Autodesk Fusion 360 part; units mm, degrees
(part 2 of 4)
  line L504 (36.7119, 7.7268) -> (35.9792, 7.7268)
  line L505 (35.9792, 7.7268) -> (35.9792, 6.8541)
  line L506 (35.9792, 6.8541) -> (37.0036, 6.8223)
  line L507 (37.0036, 6.8223) -> (37.0474, 6.7171)
  line L508 (37.0474, 6.7171) -> (36.8838, 6.6359)
  line L509 (36.8838, 6.6359) -> (35.6903, 6.6677)
  line L510 (35.6903, 6.6677) -> (35.641, 6.745)
  line L511 (7.544, 26.4091) -> (7.544, 26.4091)
  line L512 (38.6779, 6.745) -> (38.6998, 8.9814)
  line L513 (38.6998, 8.9814) -> (38.9315, 9.0218)
  line L514 (38.9315, 9.0218) -> (39.0161, 8.9268)
  line L515 (39.0161, 8.9268) -> (38.9941, 6.6904)
  line L516 (38.9941, 6.6904) -> (38.7624, 6.65)
  line L517 (38.7624, 6.65) -> (38.6779, 6.745)
  line L518 (10.5809, 26.4091) -> (10.5809, 26.4091)
  line L519 (41.4963, 7.625) -> (41.6977, 7.7268)
  line L520 (41.6977, 7.7268) -> (41.7415, 7.8359)
  line L521 (41.7415, 7.8359) -> (41.7304, 8.6571)
  line L522 (41.7304, 8.6571) -> (41.6071, 8.7735)
  line L523 (41.6071, 8.7735) -> (41.4033, 8.8177)
  line L524 (41.4033, 8.8177) -> (40.8397, 8.8177)
  line L525 (40.8397, 8.8177) -> (40.8178, 6.6904)
  line L526 (40.8178, 6.6904) -> (40.5861, 6.65)
  line L527 (40.5861, 6.65) -> (40.5015, 6.745)
  line L528 (40.5015, 6.745) -> (40.5234, 8.9814)
  line L529 (40.5234, 8.9814) -> (40.6706, 9.0359)
  line L530 (40.6706, 9.0359) -> (41.5804, 9.0217)
  line L531 (41.5804, 9.0217) -> (41.8126, 8.9469)
  line L532 (41.8126, 8.9469) -> (41.9914, 8.8165)
  line L533 (41.9914, 8.8165) -> (42.0576, 8.7138)
  line L534 (42.0576, 8.7138) -> (42.0797, 8.5995)
  line L535 (42.0797, 8.5995) -> (42.0742, 7.7774)
  line L536 (42.0742, 7.7774) -> (42.0304, 7.6691)
  line L537 (42.0304, 7.6691) -> (41.7528, 7.4614)
  line L538 (41.7528, 7.4614) -> (42.184, 6.7123)
  line L539 (42.184, 6.7123) -> (41.9726, 6.6395)
  line L540 (41.9726, 6.6395) -> (41.8711, 6.6959)
  line L541 (41.8711, 6.6959) -> (41.3709, 7.5343)
  line L542 (41.3709, 7.5343) -> (41.4963, 7.625)
  line L543 (13.3994, 27.2891) -> (13.3994, 27.2891)
  line L544 (43.4792, 7.945) -> (44.3317, 7.9132)
  line L545 (44.3317, 7.9132) -> (44.3755, 7.8071)
  line L546 (44.3755, 7.8071) -> (44.2119, 7.7268)
  line L547 (44.2119, 7.7268) -> (43.4792, 7.7268)
  line L548 (43.4792, 7.7268) -> (43.4573, 6.6904)
  line L549 (43.4573, 6.6904) -> (43.2256, 6.65)
  line L550 (43.2256, 6.65) -> (43.141, 6.745)
  line L551 (43.141, 6.745) -> (43.1629, 8.9814)
  line L552 (43.1629, 8.9814) -> (43.3101, 9.0359)
  line L553 (43.3101, 9.0359) -> (44.5036, 9.0041)
  line L554 (44.5036, 9.0041) -> (44.5474, 8.8989)
  line L555 (44.5474, 8.8989) -> (44.3838, 8.8177)
  line L556 (44.3838, 8.8177) -> (43.4792, 8.8177)
  line L557 (43.4792, 8.8177) -> (43.4792, 7.945)
  line L558 (15.3822, 27.6091) -> (15.3822, 27.6091)
  line L559 (46.1779, 8.8177) -> (45.5921, 8.8605)
  line L560 (45.5921, 8.8605) -> (45.5702, 8.9689)
  line L561 (45.5702, 8.9689) -> (45.727, 9.0359)
  line L562 (45.727, 9.0359) -> (47.0867, 9.0041)
  line L563 (47.0867, 9.0041) -> (47.1306, 8.898)
  line L564 (47.1306, 8.898) -> (46.967, 8.8177)
  line L565 (46.967, 8.8177) -> (46.5161, 8.8177)
  line L566 (46.5161, 8.8177) -> (46.4941, 6.6904)
  line L567 (46.4941, 6.6904) -> (46.2624, 6.65)
  line L568 (46.2624, 6.65) -> (46.1779, 6.745)
  line L569 (46.1779, 6.745) -> (46.1779, 8.8177)
  line L570 (18.0809, 28.4818) -> (18.0809, 28.4818)
  line L571 (48.0029, 6.745) -> (48.0248, 8.9814)
  line L572 (48.0248, 8.9814) -> (48.2566, 9.0218)
  line L573 (48.2566, 9.0218) -> (48.3411, 8.9268)
  line L574 (48.3411, 8.9268) -> (48.3411, 7.945)
  line L575 (48.3411, 7.945) -> (49.3528, 7.945)
  line L576 (49.3528, 7.945) -> (49.3747, 8.9814)
  line L577 (49.3747, 8.9814) -> (49.6065, 9.0218)
  line L578 (49.6065, 9.0218) -> (49.691, 8.9268)
  line L579 (49.691, 8.9268) -> (49.6691, 6.6904)
  line L580 (49.6691, 6.6904) -> (49.4374, 6.65)
  line L581 (49.4374, 6.65) -> (49.3528, 6.745)
  line L582 (49.3528, 6.745) -> (49.3528, 7.7268)
  line L583 (49.3528, 7.7268) -> (48.3411, 7.7268)
  line L584 (48.3411, 7.7268) -> (48.3192, 6.6904)
  line L585 (48.3192, 6.6904) -> (48.0875, 6.65)
  line L586 (48.0875, 6.65) -> (48.0029, 6.745)
  line L587 (19.906, 26.4091) -> (19.906, 26.4091)
  line L588 (51.1779, 6.745) -> (51.1998, 8.9814)
  line L589 (51.1998, 8.9814) -> (51.4315, 9.0218)
  line L590 (51.4315, 9.0218) -> (51.5161, 8.9268)
  line L591 (51.5161, 8.9268) -> (51.4941, 6.6904)
  line L592 (51.4941, 6.6904) -> (51.2624, 6.65)
  line L593 (51.2624, 6.65) -> (51.1779, 6.745)
  line L594 (23.0809, 26.4091) -> (23.0809, 26.4091)
  line L595 (53.9963, 7.625) -> (54.1977, 7.7268)
  line L596 (54.1977, 7.7268) -> (54.2415, 7.8359)
  line L597 (54.2415, 7.8359) -> (54.2304, 8.6571)
  line L598 (54.2304, 8.6571) -> (54.1071, 8.7735)
  line L599 (54.1071, 8.7735) -> (53.9033, 8.8177)
  line L600 (53.9033, 8.8177) -> (53.3397, 8.8177)
  line L601 (53.3397, 8.8177) -> (53.3178, 6.6904)
  line L602 (53.3178, 6.6904) -> (53.0861, 6.65)
  line L603 (53.0861, 6.65) -> (53.0015, 6.745)
  line L604 (53.0015, 6.745) -> (53.0234, 8.9814)
  line L605 (53.0234, 8.9814) -> (53.1706, 9.0359)
  line L606 (53.1706, 9.0359) -> (54.0804, 9.0217)
  line L607 (54.0804, 9.0217) -> (54.3126, 8.9469)
  line L608 (54.3126, 8.9469) -> (54.4914, 8.8165)
  line L609 (54.4914, 8.8165) -> (54.5576, 8.7138)
  line L610 (54.5576, 8.7138) -> (54.5797, 8.5995)
  line L611 (54.5797, 8.5995) -> (54.5742, 7.7774)
  line L612 (54.5742, 7.7774) -> (54.5304, 7.6691)
  line L613 (54.5304, 7.6691) -> (54.2528, 7.4614)
  line L614 (54.2528, 7.4614) -> (54.684, 6.7123)
  line L615 (54.684, 6.7123) -> (54.4726, 6.6395)
  line L616 (54.4726, 6.6395) -> (54.3711, 6.6959)
  line L617 (54.3711, 6.6959) -> (53.8709, 7.5343)
  line L618 (53.8709, 7.5343) -> (53.9963, 7.625)
  line L619 (25.8994, 27.2891) -> (25.8994, 27.2891)
  line L620 (56.7485, 6.9372) -> (56.9939, 6.9257)
  line L621 (56.9939, 6.9257) -> (57.0154, 6.8218)
  line L622 (57.0154, 6.8218) -> (56.9009, 6.7411)
  line L623 (56.9009, 6.7411) -> (56.6334, 6.6527)
  line L624 (56.6334, 6.6527) -> (56.3286, 6.6399)
  line L625 (56.3286, 6.6399) -> (56.0505, 6.7001)
  line L626 (56.0505, 6.7001) -> (55.8224, 6.8302)
  line L627 (55.8224, 6.8302) -> (55.7229, 6.9399)
  line L628 (55.7229, 6.9399) -> (55.6731, 7.0628)
  line L629 (55.6731, 7.0628) -> (55.6731, 8.609)
  line L630 (55.6731, 8.609) -> (55.7229, 8.7319)
  line L631 (55.7229, 8.7319) -> (55.8224, 8.8416)
  line L632 (55.8224, 8.8416) -> (56.0505, 8.9717)
  line L633 (56.0505, 8.9717) -> (56.3286, 9.0319)
  line L634 (56.3286, 9.0319) -> (56.6334, 9.0191)
  line L635 (56.6334, 9.0191) -> (56.9009, 8.9307)
  line L636 (56.9009, 8.9307) -> (57.0271, 8.8104)
  line L637 (57.0271, 8.8104) -> (56.9064, 8.7081)
  line L638 (56.9064, 8.7081) -> (56.547, 8.8131)
  line L639 (56.547, 8.8131) -> (56.2626, 8.802)
  line L640 (56.2626, 8.802) -> (56.0828, 8.7113)
  line L641 (56.0828, 8.7113) -> (56.0087, 8.6146)
  line L642 (56.0087, 8.6146) -> (55.9946, 8.5407)
  line L643 (55.9946, 8.5407) -> (55.9982, 7.0932)
  line L644 (55.9982, 7.0932) -> (56.0511, 6.9909)
  line L645 (56.0511, 6.9909) -> (56.2125, 6.8859)
  line L646 (56.2125, 6.8859) -> (56.4905, 6.8516)
  line L647 (56.4905, 6.8516) -> (56.7485, 6.9372)
  line L648 (28.6515, 26.6013) -> (28.6515, 26.6013)
  line L649 (58.141, 6.745) -> (58.1629, 8.9814)
  line L650 (58.1629, 8.9814) -> (58.3101, 9.0359)
  line L651 (58.3101, 9.0359) -> (59.5036, 9.0041)
  line L652 (59.5036, 9.0041) -> (59.5474, 8.8989)
  line L653 (59.5474, 8.8989) -> (59.3838, 8.8177)
  line L654 (59.3838, 8.8177) -> (58.4792, 8.8177)
  line L655 (58.4792, 8.8177) -> (58.4792, 7.945)
  line L656 (58.4792, 7.945) -> (59.3317, 7.9132)
  line L657 (59.3317, 7.9132) -> (59.3755, 7.8071)
  line L658 (59.3755, 7.8071) -> (59.2119, 7.7268)
  line L659 (59.2119, 7.7268) -> (58.4792, 7.7268)
  line L660 (58.4792, 7.7268) -> (58.4792, 6.8541)
  line L661 (58.4792, 6.8541) -> (59.5036, 6.8223)
  line L662 (59.5036, 6.8223) -> (59.5474, 6.7171)
  line L663 (59.5474, 6.7171) -> (59.3838, 6.6359)
  line L664 (59.3838, 6.6359) -> (58.1903, 6.6677)
  line L665 (58.1903, 6.6677) -> (58.141, 6.745)
  line L666 (30.044, 26.4091) -> (30.044, 26.4091)
  line L667 (31.9045, 5.882) -> (31.9463, 5.7785)
  line L668 (31.9463, 5.7785) -> (31.7415, 5.703)
  line L669 (31.7415, 5.703) -> (31.4641, 5.8096)
  line L670 (31.4641, 5.8096) -> (31.1753, 5.7983)
  line L671 (31.1753, 5.7983) -> (30.9927, 5.7062)
  line L672 (30.9927, 5.7062) -> (30.9175, 5.608)
  line L673 (30.9175, 5.608) -> (30.9067, 4.0986)
  line L674 (30.9067, 4.0986) -> (30.9604, 3.9946)
  line L675 (30.9604, 3.9946) -> (31.1244, 3.8881)
  line L676 (31.1244, 3.8881) -> (31.347, 3.8507)
  line L677 (31.347, 3.8507) -> (31.7908, 3.8507)
  line L678 (31.7908, 3.8507) -> (31.7908, 4.6739)
  line L679 (31.7908, 4.6739) -> (31.4795, 4.7288)
  line L680 (31.4795, 4.7288) -> (31.4795, 4.835)
  line L681 (31.4795, 4.835) -> (31.6244, 4.8887)
  line L682 (31.6244, 4.8887) -> (32.091, 4.8466)
  line L683 (32.091, 4.8466) -> (32.1237, 4.7813)
  line L684 (32.1237, 4.7813) -> (32.1021, 3.6908)
  line L685 (32.1021, 3.6908) -> (31.9573, 3.6359)
  line L686 (31.9573, 3.6359) -> (31.2423, 3.64)
  line L687 (31.2423, 3.64) -> (30.9598, 3.7007)
  line L688 (30.9598, 3.7007) -> (30.7282, 3.8321)
  line L689 (30.7282, 3.8321) -> (30.6271, 3.9431)
  line L690 (30.6271, 3.9431) -> (30.5766, 4.0677)
  line L691 (30.5766, 4.0677) -> (30.5766, 5.6023)
  line L692 (30.5766, 5.6023) -> (30.6271, 5.7272)
  line L693 (30.6271, 5.7272) -> (30.7282, 5.8385)
  line L694 (30.7282, 5.8385) -> (30.9598, 5.9707)
  line L695 (30.9598, 5.9707) -> (31.2423, 6.0318)
  line L696 (31.2423, 6.0318) -> (31.5519, 6.0188)
  line L697 (31.5519, 6.0188) -> (31.9045, 5.882)
  line L698 (3.8076, 25.5461) -> (3.8076, 25.5461)
  line L699 (33.6779, 5.8177) -> (33.0921, 5.8605)
  line L700 (33.0921, 5.8605) -> (33.0702, 5.9689)
  line L701 (33.0702, 5.9689) -> (33.227, 6.0359)
  line L702 (33.227, 6.0359) -> (34.5867, 6.0041)
  line L703 (34.5867, 6.0041) -> (34.6306, 5.898)
  line L704 (34.6306, 5.898) -> (34.467, 5.8177)
  line L705 (34.467, 5.8177) -> (34.0161, 5.8177)
  line L706 (34.0161, 5.8177) -> (33.9941, 3.6904)
  line L707 (33.9941, 3.6904) -> (33.7624, 3.65)
  line L708 (33.7624, 3.65) -> (33.6779, 3.745)
  line L709 (33.6779, 3.745) -> (33.6779, 5.8177)
  line L710 (5.5809, 25.4818) -> (5.5809, 25.4818)
  line L711 (35.7274, 5.4473) -> (35.7055, 3.6904)
  line L712 (35.7055, 3.6904) -> (35.474, 3.65)
  line L713 (35.474, 3.65) -> (35.3895, 3.7449)
  line L714 (35.3895, 3.7449) -> (35.4114, 5.9814)
  line L715 (35.4114, 5.9814) -> (35.6436, 6.0222)
  line L716 (35.6436, 6.0222) -> (35.7077, 5.9796)
  line L717 (35.7077, 5.9796) -> (36.9665, 4.2336)
  line L718 (36.9665, 4.2336) -> (36.9884, 5.9814)
  line L719 (36.9884, 5.9814) -> (37.2199, 6.0218)
  line L720 (37.2199, 6.0218) -> (37.3044, 5.9269)
  line L721 (37.3044, 5.9269) -> (37.2831, 3.6906)
  line L722 (37.2831, 3.6906) -> (37.0516, 3.6504)
  line L723 (37.0516, 3.6504) -> (36.9749, 3.7086)
  line L724 (36.9749, 3.7086) -> (35.7274, 5.4473)
  line L725 (7.6305, 25.1114) -> (7.6305, 25.1114)
  line L726 (38.9963, 4.625) -> (39.1977, 4.7268)
  line L727 (39.1977, 4.7268) -> (39.2415, 4.8359)
  line L728 (39.2415, 4.8359) -> (39.2304, 5.6571)
  line L729 (39.2304, 5.6571) -> (39.1071, 5.7735)
  line L730 (39.1071, 5.7735) -> (38.9033, 5.8177)
  line L731 (38.9033, 5.8177) -> (38.3397, 5.8177)
  line L732 (38.3397, 5.8177) -> (38.3178, 3.6904)
  line L733 (38.3178, 3.6904) -> (38.0861, 3.65)
  line L734 (38.0861, 3.65) -> (38.0015, 3.745)
  line L735 (38.0015, 3.745) -> (38.0234, 5.9814)
  line L736 (38.0234, 5.9814) -> (38.1706, 6.0359)
  line L737 (38.1706, 6.0359) -> (39.0804, 6.0217)
  line L738 (39.0804, 6.0217) -> (39.3126, 5.9469)
  line L739 (39.3126, 5.9469) -> (39.4914, 5.8165)
  line L740 (39.4914, 5.8165) -> (39.5576, 5.7138)
  line L741 (39.5576, 5.7138) -> (39.5797, 5.5995)
  line L742 (39.5797, 5.5995) -> (39.5742, 4.7774)
  line L743 (39.5742, 4.7774) -> (39.5304, 4.6691)
  line L744 (39.5304, 4.6691) -> (39.2528, 4.4614)
  line L745 (39.2528, 4.4614) -> (39.684, 3.7123)
  line L746 (39.684, 3.7123) -> (39.4726, 3.6395)
  line L747 (39.4726, 3.6395) -> (39.3711, 3.6959)
  line L748 (39.3711, 3.6959) -> (38.8709, 4.5343)
  line L749 (38.8709, 4.5343) -> (38.9963, 4.625)
  line L750 (10.8994, 24.2891) -> (10.8994, 24.2891)
  line L751 (41.1779, 5.8177) -> (40.5921, 5.8605)
  line L752 (40.5921, 5.8605) -> (40.5702, 5.9689)
  line L753 (40.5702, 5.9689) -> (40.727, 6.0359)
  line L754 (40.727, 6.0359) -> (42.0867, 6.0041)
  line L755 (42.0867, 6.0041) -> (42.1306, 5.898)
  line L756 (42.1306, 5.898) -> (41.967, 5.8177)
  line L757 (41.967, 5.8177) -> (41.5161, 5.8177)
  line L758 (41.5161, 5.8177) -> (41.4941, 3.6904)
  line L759 (41.4941, 3.6904) -> (41.2624, 3.65)
  line L760 (41.2624, 3.65) -> (41.1779, 3.745)
  line L761 (41.1779, 3.745) -> (41.1779, 5.8177)
  line L762 (13.0809, 25.4818) -> (13.0809, 25.4818)
  line L763 (43.6779, 5.8177) -> (43.0921, 5.8605)
  line L764 (43.0921, 5.8605) -> (43.0702, 5.9689)
  line L765 (43.0702, 5.9689) -> (43.227, 6.0359)
  line L766 (43.227, 6.0359) -> (44.5867, 6.0041)
  line L767 (44.5867, 6.0041) -> (44.6306, 5.898)
  line L768 (44.6306, 5.898) -> (44.467, 5.8177)
  line L769 (44.467, 5.8177) -> (44.0161, 5.8177)
  line L770 (44.0161, 5.8177) -> (43.9941, 3.6904)
  line L771 (43.9941, 3.6904) -> (43.7624, 3.65)
  line L772 (43.7624, 3.65) -> (43.6779, 3.745)
  line L773 (43.6779, 3.745) -> (43.6779, 5.8177)
  line L774 (15.5809, 25.4818) -> (15.5809, 25.4818)
  line L775 (47.8536, 5.9032) -> (47.0749, 3.6686)
  line L776 (47.0749, 3.6686) -> (46.8768, 3.6586)
  line L777 (46.8768, 3.6586) -> (46.8187, 3.7304)
  line L778 (46.8187, 3.7304) -> (46.347, 5.105)
  line L779 (46.347, 5.105) -> (45.8321, 3.6686)
  line L780 (45.8321, 3.6686) -> (45.634, 3.6586)
  line L781 (45.634, 3.6586) -> (45.5734, 3.7304)
  line L782 (45.5734, 3.7304) -> (44.8489, 5.9689)
  line L783 (44.8489, 5.9689) -> (45.049, 6.0282)
  line L784 (45.049, 6.0282) -> (45.1422, 5.945)
  line L785 (45.1422, 5.945) -> (45.7256, 4.2123)
  line L786 (45.7256, 4.2123) -> (46.2442, 5.6432)
  line L787 (46.2442, 5.6432) -> (46.4535, 5.6414)
  line L788 (46.4535, 5.6414) -> (46.5093, 5.5632)
  line L789 (46.5093, 5.5632) -> (46.9684, 4.2123)
  line L790 (46.9684, 4.2123) -> (47.5974, 6.005)
  line L791 (47.5974, 6.005) -> (47.8117, 6.0041)
  line L792 (47.8117, 6.0041) -> (47.8536, 5.9032)
  line L793 (19.7566, 25.5673) -> (19.7566, 25.5673)
  line L794 (48.141, 3.745) -> (48.1629, 5.9814)
  line L795 (48.1629, 5.9814) -> (48.3101, 6.0359)
  line L796 (48.3101, 6.0359) -> (49.5036, 6.0041)
  line L797 (49.5036, 6.0041) -> (49.5474, 5.8989)
  line L798 (49.5474, 5.8989) -> (49.3838, 5.8177)
  line L799 (49.3838, 5.8177) -> (48.4792, 5.8177)
  line L800 (48.4792, 5.8177) -> (48.4792, 4.945)
  line L801 (48.4792, 4.945) -> (49.3317, 4.9132)
  line L802 (49.3317, 4.9132) -> (49.3755, 4.8071)
  line L803 (49.3755, 4.8071) -> (49.2119, 4.7268)
  line L804 (49.2119, 4.7268) -> (48.4792, 4.7268)
  line L805 (48.4792, 4.7268) -> (48.4792, 3.8541)
  line L806 (48.4792, 3.8541) -> (49.5036, 3.8223)
  line L807 (49.5036, 3.8223) -> (49.5474, 3.7171)
  line L808 (49.5474, 3.7171) -> (49.3838, 3.6359)
  line L809 (49.3838, 3.6359) -> (48.1903, 3.6677)
  line L810 (48.1903, 3.6677) -> (48.141, 3.745)
  line L811 (20.044, 23.4091) -> (20.044, 23.4091)
  line L812 (50.7274, 5.4473) -> (50.7055, 3.6904)
  line L813 (50.7055, 3.6904) -> (50.474, 3.65)
  line L814 (50.474, 3.65) -> (50.3895, 3.7449)
  line L815 (50.3895, 3.7449) -> (50.4114, 5.9814)
  line L816 (50.4114, 5.9814) -> (50.6436, 6.0222)
  line L817 (50.6436, 6.0222) -> (50.7077, 5.9796)
  line L818 (50.7077, 5.9796) -> (51.9665, 4.2336)
  line L819 (51.9665, 4.2336) -> (51.9884, 5.9814)
  line L820 (51.9884, 5.9814) -> (52.2199, 6.0218)
  line L821 (52.2199, 6.0218) -> (52.3044, 5.9269)
  line L822 (52.3044, 5.9269) -> (52.2831, 3.6906)
  line L823 (52.2831, 3.6906) -> (52.0516, 3.6504)
  line L824 (52.0516, 3.6504) -> (51.9749, 3.7086)
  line L825 (51.9749, 3.7086) -> (50.7274, 5.4473)
  line L826 (22.6305, 25.1114) -> (22.6305, 25.1114)
  line L827 (53.6779, 5.8177) -> (53.0921, 5.8605)
  line L828 (53.0921, 5.8605) -> (53.0702, 5.9689)
  line L829 (53.0702, 5.9689) -> (53.227, 6.0359)
  line L830 (53.227, 6.0359) -> (54.5867, 6.0041)
  line L831 (54.5867, 6.0041) -> (54.6306, 5.898)
  line L832 (54.6306, 5.898) -> (54.467, 5.8177)
  line L833 (54.467, 5.8177) -> (54.0161, 5.8177)
  line L834 (54.0161, 5.8177) -> (53.9941, 3.6904)
  line L835 (53.9941, 3.6904) -> (53.7624, 3.65)
  line L836 (53.7624, 3.65) -> (53.6779, 3.745)
  line L837 (53.6779, 3.745) -> (53.6779, 5.8177)
  line L838 (25.5809, 25.4818) -> (25.5809, 25.4818)
  line L839 (56.1751, 4.3868) -> (55.5068, 5.9556)
  line L840 (55.5068, 5.9556) -> (55.6907, 6.035)
  line L841 (55.6907, 6.035) -> (55.8284, 5.9632)
  line L842 (55.8284, 5.9632) -> (56.347, 4.785)
  line L843 (56.347, 4.785) -> (56.9106, 6.005)
  line L844 (56.9106, 6.005) -> (57.1459, 6.0041)
  line L845 (57.1459, 6.0041) -> (57.184, 5.8832)
  line L846 (57.184, 5.8832) -> (56.5132, 4.385)
  line L847 (56.5132, 4.385) -> (56.4913, 3.6904)
  line L848 (56.4913, 3.6904) -> (56.2615, 3.65)
  line L849 (56.2615, 3.65) -> (56.1751, 3.745)
  line L850 (56.1751, 3.745) -> (56.1751, 4.3868)
  line L851 (28.0781, 24.0509) -> (28.0781, 24.0509)
  line L852 (58.8892, 3.8541) -> (59.1257, 3.9147)
  line L853 (59.1257, 3.9147) -> (59.2648, 4.0304)
  line L854 (59.2648, 4.0304) -> (59.2979, 4.1414)
  line L855 (59.2979, 4.1414) -> (59.2942, 5.5659)
  line L856 (59.2942, 5.5659) -> (59.239, 5.6715)
  line L857 (59.239, 5.6715) -> (59.0712, 5.7797)
  line L858 (59.0712, 5.7797) -> (58.847, 5.8177)
  line L859 (58.847, 5.8177) -> (58.3961, 5.8177)
  line L860 (58.3961, 5.8177) -> (58.3741, 3.6904)
  line L861 (58.3741, 3.6904) -> (58.1424, 3.65)
  line L862 (58.1424, 3.65) -> (58.0579, 3.745)
  line L863 (58.0579, 3.745) -> (58.0798, 5.9814)
  line L864 (58.0798, 5.9814) -> (58.227, 6.0359)
  line L865 (58.227, 6.0359) -> (58.9533, 6.0318)
  line L866 (58.9533, 6.0318) -> (59.2403, 5.9696)
  line L867 (59.2403, 5.9696) -> (59.4756, 5.8354)
  line L868 (59.4756, 5.8354) -> (59.5783, 5.7223)
  line L869 (59.5783, 5.7223) -> (59.6296, 5.5954)
  line L870 (59.6296, 5.5954) -> (59.6296, 4.0728)
  line L871 (59.6296, 4.0728) -> (59.5783, 3.9464)
  line L872 (59.5783, 3.9464) -> (59.4756, 3.834)
  line L873 (59.4756, 3.834) -> (59.259, 3.707)
  line L874 (59.259, 3.707) -> (59.0073, 3.6435)
  line L875 (59.0073, 3.6435) -> (58.7562, 3.6904)
  line L876 (58.7562, 3.6904) -> (58.7568, 3.7991)
  line L877 (58.7568, 3.7991) -> (58.8892, 3.8541)
  line L878 (30.7923, 23.5182) -> (30.7923, 23.5182)
  line L879 (31.4963, 1.625) -> (31.6977, 1.7268)
  line L880 (31.6977, 1.7268) -> (31.7415, 1.8359)
  line L881 (31.7415, 1.8359) -> (31.7304, 2.6571)
  line L882 (31.7304, 2.6571) -> (31.6071, 2.7735)
  line L883 (31.6071, 2.7735) -> (31.4033, 2.8177)
  line L884 (31.4033, 2.8177) -> (30.8397, 2.8177)
  line L885 (30.8397, 2.8177) -> (30.8178, 0.6904)
  line L886 (30.8178, 0.6904) -> (30.5861, 0.65)
  line L887 (30.5861, 0.65) -> (30.5015, 0.745)
  line L888 (30.5015, 0.745) -> (30.5234, 2.9814)
  line L889 (30.5234, 2.9814) -> (30.6706, 3.0359)
  line L890 (30.6706, 3.0359) -> (31.5804, 3.0217)
  line L891 (31.5804, 3.0217) -> (31.8126, 2.9469)
  line L892 (31.8126, 2.9469) -> (31.9914, 2.8165)
  line L893 (31.9914, 2.8165) -> (32.0576, 2.7138)
  line L894 (32.0576, 2.7138) -> (32.0797, 2.5995)
  line L895 (32.0797, 2.5995) -> (32.0742, 1.7774)
  line L896 (32.0742, 1.7774) -> (32.0304, 1.6691)
  line L897 (32.0304, 1.6691) -> (31.7528, 1.4614)
  line L898 (31.7528, 1.4614) -> (32.184, 0.7123)
  line L899 (32.184, 0.7123) -> (31.9726, 0.6395)
  line L900 (31.9726, 0.6395) -> (31.8711, 0.6959)
  line L901 (31.8711, 0.6959) -> (31.3709, 1.5343)
  line L902 (31.3709, 1.5343) -> (31.4963, 1.625)
  line L903 (3.3994, 21.2891) -> (3.3994, 21.2891)
  line L904 (33.141, 0.745) -> (33.1629, 2.9814)
  line L905 (33.1629, 2.9814) -> (33.3101, 3.0359)
  line L906 (33.3101, 3.0359) -> (34.5036, 3.0041)
  line L907 (34.5036, 3.0041) -> (34.5474, 2.8989)
  line L908 (34.5474, 2.8989) -> (34.3838, 2.8177)
  line L909 (34.3838, 2.8177) -> (33.4792, 2.8177)
  line L910 (33.4792, 2.8177) -> (33.4792, 1.945)
  line L911 (33.4792, 1.945) -> (34.3317, 1.9132)
  line L912 (34.3317, 1.9132) -> (34.3755, 1.8071)
  line L913 (34.3755, 1.8071) -> (34.2119, 1.7268)
  line L914 (34.2119, 1.7268) -> (33.4792, 1.7268)
  line L915 (33.4792, 1.7268) -> (33.4792, 0.8541)
  line L916 (33.4792, 0.8541) -> (34.5036, 0.8223)
  line L917 (34.5036, 0.8223) -> (34.5474, 0.7171)
  line L918 (34.5474, 0.7171) -> (34.3838, 0.6359)
  line L919 (34.3838, 0.6359) -> (33.1903, 0.6677)
  line L920 (33.1903, 0.6677) -> (33.141, 0.745)
  line L921 (5.044, 20.4091) -> (5.044, 20.4091)
  line L922 (36.1779, 2.8177) -> (35.5921, 2.8605)
  line L923 (35.5921, 2.8605) -> (35.5702, 2.9689)
  line L924 (35.5702, 2.9689) -> (35.727, 3.0359)
  line L925 (35.727, 3.0359) -> (37.0867, 3.0041)
  line L926 (37.0867, 3.0041) -> (37.1306, 2.898)
  line L927 (37.1306, 2.898) -> (36.967, 2.8177)
  line L928 (36.967, 2.8177) -> (36.5161, 2.8177)
  line L929 (36.5161, 2.8177) -> (36.4941, 0.6904)
  line L930 (36.4941, 0.6904) -> (36.2624, 0.65)
  line L931 (36.2624, 0.65) -> (36.1779, 0.745)
  line L932 (36.1779, 0.745) -> (36.1779, 2.8177)
  line L933 (8.0809, 22.4818) -> (8.0809, 22.4818)
  line L934 (38.6779, 2.8177) -> (38.0921, 2.8605)
  line L935 (38.0921, 2.8605) -> (38.0702, 2.9689)
  line L936 (38.0702, 2.9689) -> (38.227, 3.0359)
  line L937 (38.227, 3.0359) -> (39.5867, 3.0041)
  line L938 (39.5867, 3.0041) -> (39.6306, 2.898)
  line L939 (39.6306, 2.898) -> (39.467, 2.8177)
  line L940 (39.467, 2.8177) -> (39.0161, 2.8177)
  line L941 (39.0161, 2.8177) -> (38.9941, 0.6904)
  line L942 (38.9941, 0.6904) -> (38.7624, 0.65)
  line L943 (38.7624, 0.65) -> (38.6779, 0.745)
  line L944 (38.6779, 0.745) -> (38.6779, 2.8177)
  line L945 (10.5809, 22.4818) -> (10.5809, 22.4818)
  line L946 (41.1751, 1.3868) -> (40.5068, 2.9556)
  line L947 (40.5068, 2.9556) -> (40.6907, 3.035)
  line L948 (40.6907, 3.035) -> (40.8284, 2.9632)
  line L949 (40.8284, 2.9632) -> (41.347, 1.785)
  line L950 (41.347, 1.785) -> (41.9106, 3.005)
  line L951 (41.9106, 3.005) -> (42.1459, 3.0041)
  line L952 (42.1459, 3.0041) -> (42.184, 2.8832)
  line L953 (42.184, 2.8832) -> (41.5132, 1.385)
  line L954 (41.5132, 1.385) -> (41.4913, 0.6904)
  line L955 (41.4913, 0.6904) -> (41.2615, 0.65)
  line L956 (41.2615, 0.65) -> (41.1751, 0.745)
  line L957 (41.1751, 0.745) -> (41.1751, 1.3868)
  line L958 (13.0781, 21.0509) -> (13.0781, 21.0509)
  line L959 (43.6751, 1.3868) -> (43.0068, 2.9556)
  line L960 (43.0068, 2.9556) -> (43.1907, 3.035)
  line L961 (43.1907, 3.035) -> (43.3284, 2.9632)
  line L962 (43.3284, 2.9632) -> (43.847, 1.785)
  line L963 (43.847, 1.785) -> (44.4106, 3.005)
  line L964 (44.4106, 3.005) -> (44.6459, 3.0041)
  line L965 (44.6459, 3.0041) -> (44.684, 2.8832)
  line L966 (44.684, 2.8832) -> (44.0132, 1.385)
  line L967 (44.0132, 1.385) -> (43.9913, 0.6904)
  line L968 (43.9913, 0.6904) -> (43.7615, 0.65)
  line L969 (43.7615, 0.65) -> (43.6751, 0.745)
  line L970 (43.6751, 0.745) -> (43.6751, 1.3868)
  line L971 (15.5781, 21.0509) -> (15.5781, 21.0509)
  line L972 (45.7274, 2.4473) -> (45.7055, 0.6904)
  line L973 (45.7055, 0.6904) -> (45.474, 0.65)
  line L974 (45.474, 0.65) -> (45.3895, 0.7449)
  line L975 (45.3895, 0.7449) -> (45.4114, 2.9814)
  line L976 (45.4114, 2.9814) -> (45.6436, 3.0222)
  line L977 (45.6436, 3.0222) -> (45.7077, 2.9796)
  line L978 (45.7077, 2.9796) -> (46.9665, 1.2336)
  line L979 (46.9665, 1.2336) -> (46.9884, 2.9814)
  line L980 (46.9884, 2.9814) -> (47.2199, 3.0218)
  line L981 (47.2199, 3.0218) -> (47.3044, 2.9269)
  line L982 (47.3044, 2.9269) -> (47.2831, 0.6906)
  line L983 (47.2831, 0.6906) -> (47.0516, 0.6504)
  line L984 (47.0516, 0.6504) -> (46.9749, 0.7086)
  line L985 (46.9749, 0.7086) -> (45.7274, 2.4473)
  line L986 (17.6305, 22.1114) -> (17.6305, 22.1114)
  line L987 (48.6779, 0.745) -> (48.6998, 2.9814)
  line L988 (48.6998, 2.9814) -> (48.9315, 3.0218)
  line L989 (48.9315, 3.0218) -> (49.0161, 2.9268)
  line L990 (49.0161, 2.9268) -> (48.9941, 0.6904)
  line L991 (48.9941, 0.6904) -> (48.7624, 0.65)
  line L992 (48.7624, 0.65) -> (48.6779, 0.745)
  line L993 (20.5809, 20.4091) -> (20.5809, 20.4091)
  line L994 (50.7274, 2.4473) -> (50.7055, 0.6904)
  line L995 (50.7055, 0.6904) -> (50.474, 0.65)
  line L996 (50.474, 0.65) -> (50.3895, 0.7449)
  line L997 (50.3895, 0.7449) -> (50.4114, 2.9814)
  line L998 (50.4114, 2.9814) -> (50.6436, 3.0222)
  line L999 (50.6436, 3.0222) -> (50.7077, 2.9796)
  line L1000 (50.7077, 2.9796) -> (51.9665, 1.2336)
  line L1001 (51.9665, 1.2336) -> (51.9884, 2.9814)
  line L1002 (51.9884, 2.9814) -> (52.2199, 3.0218)
  line L1003 (52.2199, 3.0218) -> (52.3044, 2.9269)
  line L1004 (52.3044, 2.9269) -> (52.2831, 0.6906)
  line L1005 (52.2831, 0.6906) -> (52.0516, 0.6504)
  line L1006 (52.0516, 0.6504) -> (51.9749, 0.7086)
  line L1007 (51.9749, 0.7086) -> (50.7274, 2.4473)
  line L1008 (22.6305, 22.1114) -> (22.6305, 22.1114)
  line L1009 (53.141, 0.745) -> (53.1629, 2.9814)
  line L1010 (53.1629, 2.9814) -> (53.3101, 3.0359)
  line L1011 (53.3101, 3.0359) -> (54.5036, 3.0041)
  line L1012 (54.5036, 3.0041) -> (54.5474, 2.8989)
  line L1013 (54.5474, 2.8989) -> (54.3838, 2.8177)
  line L1014 (54.3838, 2.8177) -> (53.4792, 2.8177)
  line L1015 (53.4792, 2.8177) -> (53.4792, 1.945)
  line L1016 (53.4792, 1.945) -> (54.3317, 1.9132)
  line L1017 (54.3317, 1.9132) -> (54.3755, 1.8071)
  line L1018 (54.3755, 1.8071) -> (54.2119, 1.7268)
  line L1019 (54.2119, 1.7268) -> (53.4792, 1.7268)
  line L1020 (53.4792, 1.7268) -> (53.4792, 0.8541)
  line L1021 (53.4792, 0.8541) -> (54.5036, 0.8223)
  line L1022 (54.5036, 0.8223) -> (54.5474, 0.7171)
  line L1023 (54.5474, 0.7171) -> (54.3838, 0.6359)
  line L1024 (54.3838, 0.6359) -> (53.1903, 0.6677)
  line L1025 (53.1903, 0.6677) -> (53.141, 0.745)
  line L1026 (25.044, 20.4091) -> (25.044, 20.4091)
  line L1027 (55.876, 1.3583) -> (56.4819, 1.3154)
  line L1028 (56.4819, 1.3154) -> (56.5038, 1.207)
  line L1029 (56.5038, 1.207) -> (56.347, 1.1399)
  line L1030 (56.347, 1.1399) -> (55.7857, 1.1399)
  line L1031 (55.7857, 1.1399) -> (55.5657, 0.6687)
  line L1032 (55.5657, 0.6687) -> (55.3246, 0.6677)
  line L1033 (55.3246, 0.6677) -> (55.2781, 0.7687)
  line L1034 (55.2781, 0.7687) -> (56.2285, 3.0031)
  line L1035 (56.2285, 3.0031) -> (56.4508, 3.0132)
  line L1036 (56.4508, 3.0132) -> (56.5134, 2.9413)
  line L1037 (56.5134, 2.9413) -> (57.4132, 0.7163)
  line L1038 (57.4132, 0.7163) -> (57.2266, 0.6368)
  line L1039 (57.2266, 0.6368) -> (57.0802, 0.7269)
  line L1040 (57.0802, 0.7269) -> (56.347, 2.4991)
  line L1041 (56.347, 2.4991) -> (55.876, 1.3583)
  line L1042 (27.779, 21.0224) -> (27.779, 21.0224)
  line L1043 (58.0029, 0.745) -> (58.0248, 2.9814)
  line L1044 (58.0248, 2.9814) -> (58.2566, 3.0218)
  line L1045 (58.2566, 3.0218) -> (58.3411, 2.9268)
  line L1046 (58.3411, 2.9268) -> (58.3411, 1.945)
  line L1047 (58.3411, 1.945) -> (59.3528, 1.945)
  line L1048 (59.3528, 1.945) -> (59.3747, 2.9814)
  line L1049 (59.3747, 2.9814) -> (59.6065, 3.0218)
  line L1050 (59.6065, 3.0218) -> (59.691, 2.9268)
  line L1051 (59.691, 2.9268) -> (59.6691, 0.6904)
  line L1052 (59.6691, 0.6904) -> (59.4374, 0.65)
  line L1053 (59.4374, 0.65) -> (59.3528, 0.745)
  line L1054 (59.3528, 0.745) -> (59.3528, 1.7268)
  line L1055 (59.3528, 1.7268) -> (58.3411, 1.7268)
  line L1056 (58.3411, 1.7268) -> (58.3192, 0.6904)
  line L1057 (58.3192, 0.6904) -> (58.0875, 0.65)
  line L1058 (58.0875, 0.65) -> (58.0029, 0.745)
  line L1059 (29.906, 20.4091) -> (29.906, 20.4091)
  line L1060 (30.876, -1.6417) -> (31.4819, -1.6846)
  line L1061 (31.4819, -1.6846) -> (31.5038, -1.793)
  line L1062 (31.5038, -1.793) -> (31.347, -1.8601)
  line L1063 (31.347, -1.8601) -> (30.7857, -1.8601)
  line L1064 (30.7857, -1.8601) -> (30.5657, -2.3313)
  line L1065 (30.5657, -2.3313) -> (30.3246, -2.3323)
  line L1066 (30.3246, -2.3323) -> (30.2781, -2.2313)
  line L1067 (30.2781, -2.2313) -> (31.2285, 0.0031)
  line L1068 (31.2285, 0.0031) -> (31.4508, 0.0132)
  line L1069 (31.4508, 0.0132) -> (31.5134, -0.0587)
  line L1070 (31.5134, -0.0587) -> (32.4132, -2.2837)
  line L1071 (32.4132, -2.2837) -> (32.2266, -2.3632)
  line L1072 (32.2266, -2.3632) -> (32.0802, -2.2731)
  line L1073 (32.0802, -2.2731) -> (31.347, -0.5009)
  line L1074 (31.347, -0.5009) -> (30.876, -1.6417)
  line L1075 (2.779, 18.0224) -> (2.779, 18.0224)
  line L1076 (33.141, -2.255) -> (33.1629, -0.0186)
  line L1077 (33.1629, -0.0186) -> (33.3101, 0.0359)
  line L1078 (33.3101, 0.0359) -> (34.5036, 0.0041)
  line L1079 (34.5036, 0.0041) -> (34.5474, -0.1011)
  line L1080 (34.5474, -0.1011) -> (34.3838, -0.1823)
  line L1081 (34.3838, -0.1823) -> (33.4792, -0.1823)
  line L1082 (33.4792, -0.1823) -> (33.4792, -1.055)
  line L1083 (33.4792, -1.055) -> (34.3317, -1.0868)
  line L1084 (34.3317, -1.0868) -> (34.3755, -1.1929)
  line L1085 (34.3755, -1.1929) -> (34.2119, -1.2732)
  line L1086 (34.2119, -1.2732) -> (33.4792, -1.2732)
  line L1087 (33.4792, -1.2732) -> (33.4792, -2.1459)
  line L1088 (33.4792, -2.1459) -> (34.5036, -2.1777)
  line L1089 (34.5036, -2.1777) -> (34.5474, -2.2829)
  line L1090 (34.5474, -2.2829) -> (34.3838, -2.3641)
  line L1091 (34.3838, -2.3641) -> (33.1903, -2.3323)
  line L1092 (33.1903, -2.3323) -> (33.141, -2.255)
  line L1093 (5.044, 17.4091) -> (5.044, 17.4091)
  line L1094 (36.1751, -1.6132) -> (35.5068, -0.0444)
  line L1095 (35.5068, -0.0444) -> (35.6907, 0.035)
  line L1096 (35.6907, 0.035) -> (35.8284, -0.0368)
  line L1097 (35.8284, -0.0368) -> (36.347, -1.215)
  line L1098 (36.347, -1.215) -> (36.9106, 0.005)
  line L1099 (36.9106, 0.005) -> (37.1459, 0.0041)
  line L1100 (37.1459, 0.0041) -> (37.184, -0.1168)
  line L1101 (37.184, -0.1168) -> (36.5132, -1.615)
  line L1102 (36.5132, -1.615) -> (36.4913, -2.3096)
  line L1103 (36.4913, -2.3096) -> (36.2615, -2.35)
  line L1104 (36.2615, -2.35) -> (36.1751, -2.255)
  line L1105 (36.1751, -2.255) -> (36.1751, -1.6132)
  line L1106 (8.0781, 18.0509) -> (8.0781, 18.0509)
  line L1107 (38.6751, -1.6132) -> (38.0068, -0.0444)
  line L1108 (38.0068, -0.0444) -> (38.1907, 0.035)
  line L1109 (38.1907, 0.035) -> (38.3284, -0.0368)
  line L1110 (38.3284, -0.0368) -> (38.847, -1.215)
  line L1111 (38.847, -1.215) -> (39.4106, 0.005)
  line L1112 (39.4106, 0.005) -> (39.6459, 0.0041)
  line L1113 (39.6459, 0.0041) -> (39.684, -0.1168)
  line L1114 (39.684, -0.1168) -> (39.0132, -1.615)
  line L1115 (39.0132, -1.615) -> (38.9913, -2.3096)
  line L1116 (38.9913, -2.3096) -> (38.7615, -2.35)
  line L1117 (38.7615, -2.35) -> (38.6751, -2.255)
  line L1118 (38.6751, -2.255) -> (38.6751, -1.6132)
  line L1119 (10.5781, 18.0509) -> (10.5781, 18.0509)
  line L1120 (40.641, -2.255) -> (40.6629, -0.0186)
  line L1121 (40.6629, -0.0186) -> (40.8101, 0.0359)
  line L1122 (40.8101, 0.0359) -> (42.0036, 0.0041)
  line L1123 (42.0036, 0.0041) -> (42.0474, -0.1011)
  line L1124 (42.0474, -0.1011) -> (41.8838, -0.1823)
  line L1125 (41.8838, -0.1823) -> (40.9792, -0.1823)
  line L1126 (40.9792, -0.1823) -> (40.9792, -1.055)
  line L1127 (40.9792, -1.055) -> (41.8317, -1.0868)
  line L1128 (41.8317, -1.0868) -> (41.8755, -1.1929)
  line L1129 (41.8755, -1.1929) -> (41.7119, -1.2732)
  line L1130 (41.7119, -1.2732) -> (40.9792, -1.2732)
  line L1131 (40.9792, -1.2732) -> (40.9792, -2.1459)
  line L1132 (40.9792, -2.1459) -> (42.0036, -2.1777)
  line L1133 (42.0036, -2.1777) -> (42.0474, -2.2829)
  line L1134 (42.0474, -2.2829) -> (41.8838, -2.3641)
  line L1135 (41.8838, -2.3641) -> (40.6903, -2.3323)
  line L1136 (40.6903, -2.3323) -> (40.641, -2.255)
  line L1137 (12.544, 17.4091) -> (12.544, 17.4091)
  line L1138 (43.1988, -2.255) -> (43.2207, -0.0186)
  line L1139 (43.2207, -0.0186) -> (43.4524, 0.0218)
  line L1140 (43.4524, 0.0218) -> (43.537, -0.0732)
  line L1141 (43.537, -0.0732) -> (43.537, -2.1459)
  line L1142 (43.537, -2.1459) -> (44.4458, -2.1777)
  line L1143 (44.4458, -2.1777) -> (44.4897, -2.2838)
  line L1144 (44.4897, -2.2838) -> (44.3261, -2.3641)
  line L1145 (44.3261, -2.3641) -> (43.2481, -2.3323)
  line L1146 (43.2481, -2.3323) -> (43.1988, -2.255)
  line L1147 (15.1018, 17.4091) -> (15.1018, 17.4091)
  line L1148 (45.641, -2.255) -> (45.6629, -0.0186)
  line L1149 (45.6629, -0.0186) -> (45.8101, 0.0359)
  line L1150 (45.8101, 0.0359) -> (47.0036, 0.0041)
  line L1151 (47.0036, 0.0041) -> (47.0474, -0.1011)
  line L1152 (47.0474, -0.1011) -> (46.8838, -0.1823)
  line L1153 (46.8838, -0.1823) -> (45.9792, -0.1823)
  line L1154 (45.9792, -0.1823) -> (45.9792, -1.055)
  line L1155 (45.9792, -1.055) -> (46.8317, -1.0868)
  line L1156 (46.8317, -1.0868) -> (46.8755, -1.1929)
  line L1157 (46.8755, -1.1929) -> (46.7119, -1.2732)
  line L1158 (46.7119, -1.2732) -> (45.9792, -1.2732)
  line L1159 (45.9792, -1.2732) -> (45.9792, -2.1459)
  line L1160 (45.9792, -2.1459) -> (47.0036, -2.1777)
  line L1161 (47.0036, -2.1777) -> (47.0474, -2.2829)
  line L1162 (47.0474, -2.2829) -> (46.8838, -2.3641)
  line L1163 (46.8838, -2.3641) -> (45.6903, -2.3323)
  line L1164 (45.6903, -2.3323) -> (45.641, -2.255)
  line L1165 (17.544, 17.4091) -> (17.544, 17.4091)
  line L1166 (47.7789, -0.0968) -> (47.8424, 0.0138)
  line L1167 (47.8424, 0.0138) -> (48.1142, -0.055)
  line L1168 (48.1142, -0.055) -> (48.847, -1.8277)
  line L1169 (48.847, -1.8277) -> (49.6304, 0.005)
  line L1170 (49.6304, 0.005) -> (49.8686, 0.0041)
  line L1171 (49.8686, 0.0041) -> (49.9151, -0.0968)
  line L1172 (49.9151, -0.0968) -> (48.9681, -2.3314)
  line L1173 (48.9681, -2.3314) -> (48.746, -2.3414)
  line L1174 (48.746, -2.3414) -> (48.6807, -2.2696)
  line L1175 (48.6807, -2.2696) -> (47.7789, -0.0968)
  line L1176 (19.6819, 19.5673) -> (19.6819, 19.5673)
  line L1177 (50.641, -2.255) -> (50.6629, -0.0186)
  line L1178 (50.6629, -0.0186) -> (50.8101, 0.0359)
  line L1179 (50.8101, 0.0359) -> (52.0036, 0.0041)
  line L1180 (52.0036, 0.0041) -> (52.0474, -0.1011)
  line L1181 (52.0474, -0.1011) -> (51.8838, -0.1823)
  line L1182 (51.8838, -0.1823) -> (50.9792, -0.1823)
  line L1183 (50.9792, -0.1823) -> (50.9792, -1.055)
  line L1184 (50.9792, -1.055) -> (51.8317, -1.0868)
  line L1185 (51.8317, -1.0868) -> (51.8755, -1.1929)
  line L1186 (51.8755, -1.1929) -> (51.7119, -1.2732)
  line L1187 (51.7119, -1.2732) -> (50.9792, -1.2732)
  line L1188 (50.9792, -1.2732) -> (50.9792, -2.1459)
  line L1189 (50.9792, -2.1459) -> (52.0036, -2.1777)
  line L1190 (52.0036, -2.1777) -> (52.0474, -2.2829)
  line L1191 (52.0474, -2.2829) -> (51.8838, -2.3641)
  line L1192 (51.8838, -2.3641) -> (50.6903, -2.3323)
  line L1193 (50.6903, -2.3323) -> (50.641, -2.255)
  line L1194 (22.544, 17.4091) -> (22.544, 17.4091)
  line L1195 (53.2274, -0.5527) -> (53.2055, -2.3096)
  line L1196 (53.2055, -2.3096) -> (52.974, -2.35)
  line L1197 (52.974, -2.35) -> (52.8895, -2.2551)
  line L1198 (52.8895, -2.2551) -> (52.9114, -0.0186)
  line L1199 (52.9114, -0.0186) -> (53.1436, 0.0222)
  line L1200 (53.1436, 0.0222) -> (53.2077, -0.0204)
  line L1201 (53.2077, -0.0204) -> (54.4665, -1.7664)
  line L1202 (54.4665, -1.7664) -> (54.4884, -0.0186)
  line L1203 (54.4884, -0.0186) -> (54.7199, 0.0218)
  line L1204 (54.7199, 0.0218) -> (54.8044, -0.0731)
  line L1205 (54.8044, -0.0731) -> (54.7831, -2.3094)
  line L1206 (54.7831, -2.3094) -> (54.5516, -2.3496)
  line L1207 (54.5516, -2.3496) -> (54.4749, -2.2914)
  line L1208 (54.4749, -2.2914) -> (53.2274, -0.5527)
  line L1209 (25.1305, 19.1114) -> (25.1305, 19.1114)
  line L1210 (55.9792, -1.055) -> (56.8317, -1.0868)
  line L1211 (56.8317, -1.0868) -> (56.8755, -1.1929)
  line L1212 (56.8755, -1.1929) -> (56.7119, -1.2732)
  line L1213 (56.7119, -1.2732) -> (55.9792, -1.2732)
  line L1214 (55.9792, -1.2732) -> (55.9573, -2.3096)
  line L1215 (55.9573, -2.3096) -> (55.7256, -2.35)
  line L1216 (55.7256, -2.35) -> (55.641, -2.255)
  line L1217 (55.641, -2.255) -> (55.6629, -0.0186)
  line L1218 (55.6629, -0.0186) -> (55.8101, 0.0359)
  line L1219 (55.8101, 0.0359) -> (57.0036, 0.0041)
  line L1220 (57.0036, 0.0041) -> (57.0474, -0.1011)
  line L1221 (57.0474, -0.1011) -> (56.8838, -0.1823)
  line L1222 (56.8838, -0.1823) -> (55.9792, -0.1823)
  line L1223 (55.9792, -0.1823) -> (55.9792, -1.055)
  line L1224 (27.8822, 18.6091) -> (27.8822, 18.6091)
  line L1225 (58.0691, -1.8622) -> (58.0907, -0.0179)
  line L1226 (58.0907, -0.0179) -> (58.3191, 0.022)
  line L1227 (58.3191, 0.022) -> (58.4025, -0.0716)
  line L1228 (58.4025, -0.0716) -> (58.4061, -1.9007)
  line L1229 (58.4061, -1.9007) -> (58.4605, -2.0048)
  line L1230 (58.4605, -2.0048) -> (58.6259, -2.1116)
  line L1231 (58.6259, -2.1116) -> (58.9066, -2.1467)
  line L1232 (58.9066, -2.1467) -> (59.1159, -2.0905)
  line L1233 (59.1159, -2.0905) -> (59.2588, -1.972)
  line L1234 (59.2588, -1.972) -> (59.2915, -1.8622)
  line L1235 (59.2915, -1.8622) -> (59.3131, -0.0179)
  line L1236 (59.3131, -0.0179) -> (59.5415, 0.022)
  line L1237 (59.5415, 0.022) -> (59.6249, -0.0716)
  line L1238 (59.6249, -0.0716) -> (59.6185, -1.9298)
  line L1239 (59.6185, -1.9298) -> (59.5679, -2.0549)
  line L1240 (59.5679, -2.0549) -> (59.4667, -2.1664)
  line L1241 (59.4667, -2.1664) -> (59.2347, -2.2988)
  line L1242 (59.2347, -2.2988) -> (58.9518, -2.36)
  line L1243 (58.9518, -2.36) -> (58.6426, -2.3478)
  line L1244 (58.6426, -2.3478) -> (58.3754, -2.262)
  line L1245 (58.3754, -2.262) -> (58.2273, -2.1664)
  line L1246 (58.2273, -2.1664) -> (58.126, -2.0549)
  line L1247 (58.126, -2.0549) -> (58.0691, -1.8622)
  line L1248 (29.9721, 17.8019) -> (29.9721, 17.8019)
  line L1249 (31.7485, -5.0628) -> (31.9939, -5.0743)
  line L1250 (31.9939, -5.0743) -> (32.0154, -5.1782)
  line L1251 (32.0154, -5.1782) -> (31.9009, -5.2589)
  line L1252 (31.9009, -5.2589) -> (31.6334, -5.3473)
  line L1253 (31.6334, -5.3473) -> (31.3286, -5.3601)
  line L1254 (31.3286, -5.3601) -> (31.0505, -5.2999)
  line L1255 (31.0505, -5.2999) -> (30.8224, -5.1698)
  line L1256 (30.8224, -5.1698) -> (30.7229, -5.0601)
  line L1257 (30.7229, -5.0601) -> (30.6731, -4.9372)
  line L1258 (30.6731, -4.9372) -> (30.6731, -3.391)
  line L1259 (30.6731, -3.391) -> (30.7229, -3.2681)
  line L1260 (30.7229, -3.2681) -> (30.8224, -3.1584)
  line L1261 (30.8224, -3.1584) -> (31.0505, -3.0283)
  line L1262 (31.0505, -3.0283) -> (31.3286, -2.9681)
  line L1263 (31.3286, -2.9681) -> (31.6334, -2.9809)
  line L1264 (31.6334, -2.9809) -> (31.9009, -3.0693)
  line L1265 (31.9009, -3.0693) -> (32.0271, -3.1896)
  line L1266 (32.0271, -3.1896) -> (31.9064, -3.2919)
  line L1267 (31.9064, -3.2919) -> (31.547, -3.1869)
  line L1268 (31.547, -3.1869) -> (31.2626, -3.198)
  line L1269 (31.2626, -3.198) -> (31.0828, -3.2887)
  line L1270 (31.0828, -3.2887) -> (31.0087, -3.3854)
  line L1271 (31.0087, -3.3854) -> (30.9946, -3.4593)
  line L1272 (30.9946, -3.4593) -> (30.9982, -4.9068)
  line L1273 (30.9982, -4.9068) -> (31.0511, -5.0091)
  line L1274 (31.0511, -5.0091) -> (31.2125, -5.1141)
  line L1275 (31.2125, -5.1141) -> (31.4905, -5.1484)
  line L1276 (31.4905, -5.1484) -> (31.7485, -5.0628)
  line L1277 (3.6515, 14.6013) -> (3.6515, 14.6013)
  line L1278 (33.2274, -3.5527) -> (33.2055, -5.3096)
  line L1279 (33.2055, -5.3096) -> (32.974, -5.35)
  line L1280 (32.974, -5.35) -> (32.8895, -5.2551)
  line L1281 (32.8895, -5.2551) -> (32.9114, -3.0186)
  line L1282 (32.9114, -3.0186) -> (33.1436, -2.9778)
  line L1283 (33.1436, -2.9778) -> (33.2077, -3.0204)
  line L1284 (33.2077, -3.0204) -> (34.4665, -4.7664)
  line L1285 (34.4665, -4.7664) -> (34.4884, -3.0186)
  line L1286 (34.4884, -3.0186) -> (34.7199, -2.9782)
  line L1287 (34.7199, -2.9782) -> (34.8044, -3.0731)
  line L1288 (34.8044, -3.0731) -> (34.7831, -5.3094)
  line L1289 (34.7831, -5.3094) -> (34.5516, -5.3496)
  line L1290 (34.5516, -5.3496) -> (34.4749, -5.2914)
  line L1291 (34.4749, -5.2914) -> (33.2274, -3.5527)
  line L1292 (5.1305, 16.1114) -> (5.1305, 16.1114)
  line L1293 (36.1779, -3.1823) -> (35.5921, -3.1395)
  line L1294 (35.5921, -3.1395) -> (35.5702, -3.0311)
  line L1295 (35.5702, -3.0311) -> (35.727, -2.9641)
  line L1296 (35.727, -2.9641) -> (37.0867, -2.9959)
  line L1297 (37.0867, -2.9959) -> (37.1306, -3.102)
  line L1298 (37.1306, -3.102) -> (36.967, -3.1823)
  line L1299 (36.967, -3.1823) -> (36.5161, -3.1823)
  line L1300 (36.5161, -3.1823) -> (36.4941, -5.3096)
  line L1301 (36.4941, -5.3096) -> (36.2624, -5.35)
  line L1302 (36.2624, -5.35) -> (36.1779, -5.255)
  line L1303 (36.1779, -5.255) -> (36.1779, -3.1823)
  line L1304 (8.0809, 16.4818) -> (8.0809, 16.4818)
  line L1305 (40.3536, -3.0968) -> (39.5749, -5.3314)
  line L1306 (39.5749, -5.3314) -> (39.3768, -5.3414)
  line L1307 (39.3768, -5.3414) -> (39.3187, -5.2696)
  line L1308 (39.3187, -5.2696) -> (38.847, -3.895)
  line L1309 (38.847, -3.895) -> (38.3321, -5.3314)
  line L1310 (38.3321, -5.3314) -> (38.134, -5.3414)
  line L1311 (38.134, -5.3414) -> (38.0734, -5.2696)
  line L1312 (38.0734, -5.2696) -> (37.3489, -3.0311)
  line L1313 (37.3489, -3.0311) -> (37.549, -2.9718)
  line L1314 (37.549, -2.9718) -> (37.6422, -3.055)
  line L1315 (37.6422, -3.055) -> (38.2256, -4.7877)
  line L1316 (38.2256, -4.7877) -> (38.7442, -3.3568)
  line L1317 (38.7442, -3.3568) -> (38.9535, -3.3586)
  line L1318 (38.9535, -3.3586) -> (39.0093, -3.4368)
  line L1319 (39.0093, -3.4368) -> (39.4684, -4.7877)
  line L1320 (39.4684, -4.7877) -> (40.0974, -2.995)
  line L1321 (40.0974, -2.995) -> (40.3117, -2.9959)
  line L1322 (40.3117, -2.9959) -> (40.3536, -3.0968)
  line L1323 (12.2566, 16.5673) -> (12.2566, 16.5673)
  line L1324 (40.641, -5.255) -> (40.6629, -3.0186)
  line L1325 (40.6629, -3.0186) -> (40.8101, -2.9641)
  line L1326 (40.8101, -2.9641) -> (42.0036, -2.9959)
  line L1327 (42.0036, -2.9959) -> (42.0474, -3.1011)
  line L1328 (42.0474, -3.1011) -> (41.8838, -3.1823)
  line L1329 (41.8838, -3.1823) -> (40.9792, -3.1823)
  line L1330 (40.9792, -3.1823) -> (40.9792, -4.055)
  line L1331 (40.9792, -4.055) -> (41.8317, -4.0868)
  line L1332 (41.8317, -4.0868) -> (41.8755, -4.1929)
  line L1333 (41.8755, -4.1929) -> (41.7119, -4.2732)
  line L1334 (41.7119, -4.2732) -> (40.9792, -4.2732)
  line L1335 (40.9792, -4.2732) -> (40.9792, -5.1459)
  line L1336 (40.9792, -5.1459) -> (42.0036, -5.1777)
  line L1337 (42.0036, -5.1777) -> (42.0474, -5.2829)
  line L1338 (42.0474, -5.2829) -> (41.8838, -5.3641)
  line L1339 (41.8838, -5.3641) -> (40.6903, -5.3323)
  line L1340 (40.6903, -5.3323) -> (40.641, -5.255)
  line L1341 (12.544, 14.4091) -> (12.544, 14.4091)
  line L1342 (43.1988, -5.255) -> (43.2207, -3.0186)
  line L1343 (43.2207, -3.0186) -> (43.4524, -2.9782)
  line L1344 (43.4524, -2.9782) -> (43.537, -3.0732)
  line L1345 (43.537, -3.0732) -> (43.537, -5.1459)
  line L1346 (43.537, -5.1459) -> (44.4458, -5.1777)
  line L1347 (44.4458, -5.1777) -> (44.4897, -5.2838)
  line L1348 (44.4897, -5.2838) -> (44.3261, -5.3641)
  line L1349 (44.3261, -5.3641) -> (43.2481, -5.3323)
  line L1350 (43.2481, -5.3323) -> (43.1988, -5.255)
  line L1351 (15.1018, 14.4091) -> (15.1018, 14.4091)
  line L1352 (45.2789, -3.0968) -> (45.3424, -2.9862)
  line L1353 (45.3424, -2.9862) -> (45.6142, -3.055)
  line L1354 (45.6142, -3.055) -> (46.347, -4.8277)
  line L1355 (46.347, -4.8277) -> (47.1304, -2.995)
  line L1356 (47.1304, -2.995) -> (47.3686, -2.9959)
  line L1357 (47.3686, -2.9959) -> (47.4151, -3.0968)
  line L1358 (47.4151, -3.0968) -> (46.4681, -5.3314)
  line L1359 (46.4681, -5.3314) -> (46.1852, -5.2809)
  line L1360 (46.1852, -5.2809) -> (45.2789, -3.0968)
  line L1361 (17.1819, 16.5673) -> (17.1819, 16.5673)
  line L1362 (48.141, -5.255) -> (48.1629, -3.0186)
  line L1363 (48.1629, -3.0186) -> (48.3101, -2.9641)
  line L1364 (48.3101, -2.9641) -> (49.5036, -2.9959)
  line L1365 (49.5036, -2.9959) -> (49.5474, -3.1011)
  line L1366 (49.5474, -3.1011) -> (49.3838, -3.1823)
  line L1367 (49.3838, -3.1823) -> (48.4792, -3.1823)
  line L1368 (48.4792, -3.1823) -> (48.4792, -4.055)
  line L1369 (48.4792, -4.055) -> (49.3317, -4.0868)
  line L1370 (49.3317, -4.0868) -> (49.3755, -4.1929)
  line L1371 (49.3755, -4.1929) -> (49.2119, -4.2732)
  line L1372 (49.2119, -4.2732) -> (48.4792, -4.2732)
  line L1373 (48.4792, -4.2732) -> (48.4792, -5.1459)
  line L1374 (48.4792, -5.1459) -> (49.5036, -5.1777)
  line L1375 (49.5036, -5.1777) -> (49.5474, -5.2829)
  line L1376 (49.5474, -5.2829) -> (49.3838, -5.3641)
  line L1377 (49.3838, -5.3641) -> (48.1903, -5.3323)
  line L1378 (48.1903, -5.3323) -> (48.141, -5.255)
  line L1379 (20.044, 14.4091) -> (20.044, 14.4091)
  line L1380 (51.9797, -4.8444) -> (51.771, -4.9159)
  line L1381 (51.771, -4.9159) -> (51.6925, -4.7346)
  line L1382 (51.6925, -4.7346) -> (51.6793, -3.3544)
  line L1383 (51.6793, -3.3544) -> (51.5731, -3.2379)
  line L1384 (51.5731, -3.2379) -> (51.3405, -3.163)
  line L1385 (51.3405, -3.163) -> (51.0838, -3.1951)
  line L1386 (51.0838, -3.1951) -> (50.9325, -3.2927)
  line L1387 (50.9325, -3.2927) -> (50.8827, -3.3879)
  line L1388 (50.8827, -3.3879) -> (50.8917, -4.802)
  line L1389 (50.8917, -4.802) -> (50.99, -4.9084)
  line L1390 (50.99, -4.9084) -> (52.1118, -5.2969)
  line L1391 (52.1118, -5.2969) -> (51.9161, -5.3592)
  line L1392 (51.9161, -5.3592) -> (50.8724, -5.106)
  line L1393 (50.8724, -5.106) -> (50.7192, -5.0128)
  line L1394 (50.7192, -5.0128) -> (50.6266, -4.9108)
  line L1395 (50.6266, -4.9108) -> (50.5803, -4.7964)
  line L1396 (50.5803, -4.7964) -> (50.5803, -3.3613)
  line L1397 (50.5803, -3.3613) -> (50.6266, -3.2469)
  line L1398 (50.6266, -3.2469) -> (50.7192, -3.1449)
  line L1399 (50.7192, -3.1449) -> (50.9314, -3.0238)
  line L1400 (50.9314, -3.0238) -> (51.1901, -2.9678)
  line L1401 (51.1901, -2.9678) -> (51.4729, -2.979)
  line L1402 (51.4729, -2.979) -> (51.7172, -3.0575)
  line L1403 (51.7172, -3.0575) -> (51.9049, -3.1943)
  line L1404 (51.9049, -3.1943) -> (51.9743, -3.3025)
  line L1405 (51.9743, -3.3025) -> (51.9975, -3.4231)
  line L1406 (51.9975, -3.4231) -> (51.9797, -4.8444)
  line L1407 (23.8827, 14.8197) -> (23.8827, 14.8197)
  line L1408 (54.2471, -3.1823) -> (53.079, -3.1505)
  line L1409 (53.079, -3.1505) -> (53.0352, -3.0444)
  line L1410 (53.0352, -3.0444) -> (53.1988, -2.9641)
  line L1411 (53.1988, -2.9641) -> (54.6149, -2.9959)
  line L1412 (54.6149, -2.9959) -> (54.653, -3.115)
  line L1413 (54.653, -3.115) -> (53.4468, -5.1459)
  line L1414 (53.4468, -5.1459) -> (54.6149, -5.1777)
  line L1415 (54.6149, -5.1777) -> (54.6588, -5.2829)
  line L1416 (54.6588, -5.2829) -> (54.4951, -5.3641)
  line L1417 (54.4951, -5.3641) -> (53.0818, -5.3314)
  line L1418 (53.0818, -5.3314) -> (53.0466, -5.2059)
  line L1419 (53.0466, -5.2059) -> (54.2471, -3.1823)
  line L1420 (26.1502, 16.4818) -> (26.1502, 16.4818)
  line L1421 (56.1779, -5.255) -> (56.1998, -3.0186)
  line L1422 (56.1998, -3.0186) -> (56.4315, -2.9782)
  line L1423 (56.4315, -2.9782) -> (56.5161, -3.0732)
  line L1424 (56.5161, -3.0732) -> (56.4941, -5.3096)
  line L1425 (56.4941, -5.3096) -> (56.2624, -5.35)
  line L1426 (56.2624, -5.35) -> (56.1779, -5.255)
  line L1427 (28.0809, 14.4091) -> (28.0809, 14.4091)
  line L1428 (58.2274, -3.5527) -> (58.2055, -5.3096)
  line L1429 (58.2055, -5.3096) -> (57.974, -5.35)
  line L1430 (57.974, -5.35) -> (57.8895, -5.2551)
  line L1431 (57.8895, -5.2551) -> (57.9114, -3.0186)
  line L1432 (57.9114, -3.0186) -> (58.1436, -2.9778)
  line L1433 (58.1436, -2.9778) -> (58.2077, -3.0204)
  line L1434 (58.2077, -3.0204) -> (59.4665, -4.7664)
  line L1435 (59.4665, -4.7664) -> (59.4884, -3.0186)
  line L1436 (59.4884, -3.0186) -> (59.7199, -2.9782)
  line L1437 (59.7199, -2.9782) -> (59.8044, -3.0731)
  line L1438 (59.8044, -3.0731) -> (59.7831, -5.3094)
  line L1439 (59.7831, -5.3094) -> (59.5516, -5.3496)
  line L1440 (59.5516, -5.3496) -> (59.4749, -5.2914)
  line L1441 (59.4749, -5.2914) -> (58.2274, -3.5527)
  line L1442 (30.1305, 16.1114) -> (30.1305, 16.1114)
  line L1443 (30.641, -8.255) -> (30.6629, -6.0186)
  line L1444 (30.6629, -6.0186) -> (30.8101, -5.9641)
  line L1445 (30.8101, -5.9641) -> (32.0036, -5.9959)
  line L1446 (32.0036, -5.9959) -> (32.0474, -6.1011)
  line L1447 (32.0474, -6.1011) -> (31.8838, -6.1823)
  line L1448 (31.8838, -6.1823) -> (30.9792, -6.1823)
  line L1449 (30.9792, -6.1823) -> (30.9792, -7.055)
  line L1450 (30.9792, -7.055) -> (31.8317, -7.0868)
  line L1451 (31.8317, -7.0868) -> (31.8755, -7.1929)
  line L1452 (31.8755, -7.1929) -> (31.7119, -7.2732)
  line L1453 (31.7119, -7.2732) -> (30.9792, -7.2732)
  line L1454 (30.9792, -7.2732) -> (30.9792, -8.1459)
  line L1455 (30.9792, -8.1459) -> (32.0036, -8.1777)
  line L1456 (32.0036, -8.1777) -> (32.0474, -8.2829)
  line L1457 (32.0474, -8.2829) -> (31.8838, -8.3641)
  line L1458 (31.8838, -8.3641) -> (30.6903, -8.3323)
  line L1459 (30.6903, -8.3323) -> (30.641, -8.255)
  line L1460 (2.544, 11.4091) -> (2.544, 11.4091)
  line L1461 (33.6779, -6.1823) -> (33.0921, -6.1395)
  line L1462 (33.0921, -6.1395) -> (33.0702, -6.0311)
  line L1463 (33.0702, -6.0311) -> (33.227, -5.9641)
  line L1464 (33.227, -5.9641) -> (34.5867, -5.9959)
  line L1465 (34.5867, -5.9959) -> (34.6306, -6.102)
  line L1466 (34.6306, -6.102) -> (34.467, -6.1823)
  line L1467 (34.467, -6.1823) -> (34.0161, -6.1823)
  line L1468 (34.0161, -6.1823) -> (33.9941, -8.3096)